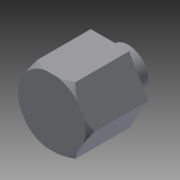
# Autodesk Inventor part: 13_5_CylinderBase
Saved by Autodesk Inventor 2015 (Build 190159000, 159)
## iProperties
Created: 2015-04-01
Part Number: 13_5_CylinderBase
Material: Generic
Document SubType Name: Modeling
Designer: WASHHSST
Density: 1 g/cm^3
Appearance: Default
Author: WASHHSST
Autodesk Inventor part; units mm, degrees
ref_plane "YZ Plane" through (0, 0, 0) normal (1, 0, 0) x (0, 1, 0)
ref_plane "XZ Plane" through (0, 0, 0) normal (0, 1, 0) x (-1, 0, 0)
ref_plane "XY Plane" through (0, 0, 0) normal (0, 0, 1) x (1, 0, 0)
sketch "Sketch1" plane through (0, 0, 0) normal (0, 0, 1) x (1, 0, 0)
  circle A0 centre (0, 0) radius 6.35
  dimension "d0" = 12.7
  constraints: 1 centre point, 1 coincident
  measures "d0" diameter of A0
extrude "Extrusion1" add sketch "Sketch1" along normal blind 9.652
sketch "Sketch2" plane through (0, 0, 0) normal (0, 0, -1) x (-1, 0, 0)
  circle A0 centre (0, 0) radius 3.302
  dimension "d3" = 6.604
  constraints: 1 centre point, 1 coincident
  measures "d3" diameter of A0
extrude "Extrusion2" add sketch "Sketch2" along normal blind 3.048
chamfer "Chamfer1" distance 0.762 angle 45 1 edges at (-6.35, 0, 9.652) measured on face at (-1.8127, -0.4771, 9.652)
sketch "Sketch3" plane through (0, 0, 9.652) normal (0, 0, 1) x (1, 0, 0)
  circle A0 centre (0, 0) radius 6.35 projected
  line L0 (3.175, 5.4993) -> (6.35, 0)
  line L1 (6.35, 0) -> (3.175, -5.4993)
  line L2 (3.175, -5.4993) -> (-3.175, -5.4993)
  line L3 (-3.175, -5.4993) -> (-6.35, 0)
  line L4 (-6.35, 0) -> (-3.175, 5.4993)
  line L5 (-3.175, 5.4993) -> (3.175, 5.4993)
  line L6 (-10.603, 0.0515) -> (9.8262, 0.0515) construction
  constraints: 14 end point, 1 coincident, 1 horizontal, 1 parallel, 15 other
extrude "Extrusion3" cut sketch "Sketch3" against normal up to surface (9.652 mm away) contours L0 A0 | A0 L1 | L5 A0 | A0 L2 | L4 A0 | A0 L3
sketch "Sketch5" plane through (0, 0, -3.048) normal (0, 0, -1) x (-1, 0, 0)
  circle A0 centre (0, 0) radius 3.937
  dimension "d15" = 7.874
  constraints: 1 centre point, 1 coincident
  measures "d15" diameter of A0
extrude "Extrusion5" [suppressed]
chamfer "Chamfer2" [suppressed]
thread "Thread1"
sketch "Sketch6" plane through (-3.175, 5.4993, 11.0682) normal (0, 1, 0) x (1, 0, 0)
  line L0 (0, 0) -> (0, 9.652)
  line L1 (0, 7.7662) -> (6.35, 7.7662)
  line L2 (6.35, 0) -> (6.35, 9.652)
  line L3 (-0.762, 14.1162) -> (7.112, 14.1162)
  line L4 (-0.762, 14.1162) -> (7.112, 14.1162) projected
  point P0 (3.175, 0)
  point P1 (3.175, 7.7662)
  dimension "d25" = 6.35
  dimension "d36" = 6.35
  dimension "d37" = 3.175
  dimension "d45" = 0
  constraints: 8 end point, 2 point on line, 1 horizontal, 1 midpoint
  measures "d25" distance between parallel lines of L1 L3
  measures "d36" distance between parallel lines of L2 L0
  measures "d37" distance from line of point (3.175, 7.766) L0
  measures "d45" distance between parallel lines of L4 L3
hole "Hole1" [suppressed]
pattern_circular "Circular Pattern1" [suppressed]
sketch "Sketch7" plane through (0, 0, 9.652) normal (0, 0, 1) x (1, 0, 0)
  point P0 (0, 0)
  point P1 (0, 0)
  constraints: 1 coincident
hole "Hole2" [suppressed]
body "Solid1"
